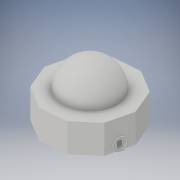
# Autodesk Inventor part: dome
Saved by Autodesk Inventor 2017 (Build 210142000, 142)
## iProperties
Created: 2018-03-05
Part Number: dome
Material: Generic
Document SubType Name: Modeling
Designer: Braxton
Density: 1 g/cm^3
Appearance: Default
Author: Braxton
Autodesk Inventor part; units mm, degrees
ref_plane "YZ Plane" through (0, 0, 0) normal (1, 0, 0) x (0, 1, 0)
sketch "Sketch1" plane through (0, 0, 0) normal (0, 1, 0) x (-1, 0, 0)
  line L0 (707.6587, -429.7359) -> (319.9155, -763.615)
  line L1 (319.9155, -763.615) -> (-190.0245, -805.8191)
  line L2 (-190.0245, -805.8191) -> (-627.3817, -540.2278)
  line L3 (-627.3817, -540.2278) -> (-825.1003, -68.2877)
  line L4 (-825.1003, -68.2877) -> (-707.6587, 429.7359)
  line L5 (-707.6587, 429.7359) -> (-319.9155, 763.615)
  line L6 (-319.9155, 763.615) -> (190.0245, 805.8191)
  line L7 (190.0245, 805.8191) -> (627.3817, 540.2278)
  line L8 (627.3817, 540.2278) -> (825.1003, 68.2877)
  line L9 (825.1003, 68.2877) -> (707.6587, -429.7359)
  point P0 (0, 0)
  point P1 (0, 0)
  dimension "d0" = 1574.8
  constraints: 20 end point, 1 coincident, 21 other
  measures "d0" distance between parallel lines of L5 L0
extrude "bace" add sketch "Sketch1" along normal blind 25.4
sketch "Sketch2" plane through (0, 25.4, 0) normal (0, 1, 0) x (1, 0, 0)
  line L0 (-319.9155, 763.615) -> (-707.6587, 429.7359) projected
  line L1 (-707.6587, 429.7359) -> (-319.9155, 763.615)
  line L2 (-319.9155, 763.615) -> (190.0245, 805.8191)
  line L3 (190.0245, 805.8191) -> (627.3817, 540.2278)
  line L4 (627.3817, 540.2278) -> (825.1003, 68.2877)
  line L5 (825.1003, 68.2877) -> (707.6587, -429.7359)
  line L6 (707.6587, -429.7359) -> (319.9155, -763.615)
  line L7 (319.9155, -763.615) -> (-190.0245, -805.8191)
  line L8 (-190.0245, -805.8191) -> (-627.3817, -540.2278)
  line L9 (-627.3817, -540.2278) -> (-825.1003, -68.2877)
  line L10 (-825.1003, -68.2877) -> (-707.6587, 429.7359)
  line L11 (-684.831, 415.8734) -> (-309.5957, 738.9822)
  line L12 (-309.5957, 738.9822) -> (183.8947, 779.825)
  line L13 (183.8947, 779.825) -> (607.1435, 522.8011)
  line L14 (607.1435, 522.8011) -> (798.4842, 66.0849)
  line L15 (798.4842, 66.0849) -> (684.831, -415.8734)
  line L16 (684.831, -415.8734) -> (309.5957, -738.9822)
  line L17 (309.5957, -738.9822) -> (-183.8947, -779.825)
  line L18 (-183.8947, -779.825) -> (-607.1435, -522.8011)
  line L19 (-607.1435, -522.8011) -> (-798.4842, -66.0849)
  line L20 (-798.4842, -66.0849) -> (-684.831, 415.8734)
  line L21 (-707.6587, 429.7359) -> (-825.1003, -68.2877) projected
  point P0 (0, 0)
  point P1 (0, 0)
  point P2 (0, 0)
  dimension "d4" = 25.4
  constraints: 40 end point, 2 coincident, 1 parallel, 42 other
  measures "d4" distance between parallel lines of L21 L20
extrude "bace wall" add sketch "Sketch2" along normal blind 508
sketch "Sketch3" plane through (0, 533.4, 0) normal (0, 1, 0) x (1, 0, 0)
  line L0 (-627.3817, -540.2278) -> (-825.1003, -68.2877) projected
  line L1 (-825.1003, -68.2877) -> (-707.6587, 429.7359)
  line L2 (-707.6587, 429.7359) -> (-319.9155, 763.615)
  line L3 (-319.9155, 763.615) -> (190.0245, 805.8191)
  line L4 (190.0245, 805.8191) -> (627.3817, 540.2278)
  line L5 (627.3817, 540.2278) -> (825.1003, 68.2877)
  line L6 (825.1003, 68.2877) -> (707.6587, -429.7359)
  line L7 (707.6587, -429.7359) -> (319.9155, -763.615)
  line L8 (319.9155, -763.615) -> (-190.0245, -805.8191)
  line L9 (-190.0245, -805.8191) -> (-627.3817, -540.2278)
  line L10 (-627.3817, -540.2278) -> (-825.1003, -68.2877)
  circle A0 centre (0, 0) radius 508
  point P0 (-798.4842, -66.0849)
  dimension "d28" = 1016
  constraints: 20 end point, 1 centre point
  measures "d28" diameter of A0
extrude "bace cieiling" add sketch "Sketch3" along normal blind 25.4
ref_plane "dome work plane" through (56.8266, 25.4, -240.9792) normal (0.9733039, 0, 0.22952) x (0.22952, 0, -0.9733039)
sketch "Sketch10" plane through (56.8266, 25.4, -240.9792) normal (0.9733039, 0, 0.22952) x (0.22952, 0, -0.9733039)
  line L0 (285.8112, 533.4) -> (260.4112, 533.4)
  line L1 (-755.5888, 533.4) -> (260.4112, 533.4) projected
  arc A0 (260.4112, 533.4) -> (-247.5888, 1041.4) centre (-247.5888, 533.4) ccw
  arc A1 (285.8112, 533.4) -> (-247.5888, 1066.8) centre (-247.5888, 533.4) ccw
  line L2 (-247.5888, 1066.8) -> (-247.5888, 1041.4)
  line L3 (-247.5888, 1041.4) -> (-247.5888, 533.4) construction
  point P0 (-247.5888, -25.4)
  dimension "d32" = 508
  dimension "d33" = 533.4
  constraints: 6 end point, 4 point on circle, 2 centre point, 2 coincident, 2 vertical, 1 midpoint
  measures "d32" radius of A0
  measures "d33" radius of A1
revolve "dome" add sketch "Sketch10" angle 360 about axis through (0, 1066.8, 0) along (0, -1, 0)
sketch "Sketch8" plane through (825.1003, 0, -68.2877) normal (0.9733039, 0, 0.22952) x (0.22952, 0, -0.9733039)
  line L0 (-255.8418, 25.4) -> (-205.0418, 25.4)
  line L1 (-205.0418, 25.4) -> (-205.0418, 194.7333)
  line L2 (-205.0418, 194.7333) -> (-255.8418, 194.7333)
  line L3 (-255.8418, 194.7333) -> (-255.8418, 25.4)
  line L4 (-255.8418, 25.4) -> (-306.6418, 25.4)
  line L5 (-306.6418, 25.4) -> (-306.6418, 194.7333)
  line L6 (-306.6418, 194.7333) -> (-255.8418, 194.7333)
  line L7 (-503.4306, 25.4) -> (-8.253, 25.4) projected
  point P0 (-255.8418, 0)
  point P1 (-255.8418, 25.4)
  dimension "d16" = 50.8
  dimension "d17" = 169.3333
  constraints: 14 end point, 2 symmetric about line, 1 horizontal, 1 midpoint, 1 perpendicular
  measures "d16" distance of L0.start L0.end
  measures "d17" distance of L0.end L1.end
extrude "door frame" cut sketch "Sketch8" against normal blind 25.4
sketch "Sketch7" plane through (825.1003, 0, -68.2877) normal (0.9733039, 0, 0.22952) x (0.22952, 0, -0.9733039)
  line L0 (-306.6418, 194.7333) -> (-205.0418, 194.7333)
  line L1 (-306.6418, 25.4) -> (-205.0418, 25.4)
  arc A0 (-198.4359, 0) -> (-313.6926, 0.2332) centre (-255.8418, 110.0667) ccw
  arc A1 (-306.6418, 194.7333) -> (-306.6418, 25.4) centre (-255.8418, 110.0667) ccw
  arc A2 (-205.0418, 25.4) -> (-205.0418, 194.7333) centre (-255.8418, 110.0667) ccw
  line L2 (-306.6418, 194.7333) -> (-205.0418, 194.7333)
  line L3 (-306.6418, 194.7333) -> (-306.6418, 25.4)
  line L4 (-313.6926, 0.2332) -> (-198.4359, 0)
  point P0 (-255.8418, 0)
  point P1 (-255.8418, 194.7333)
  point P2 (-306.6418, 110.0667)
  point P3 (-255.8418, 110.0667)
  point P4 (-256.0642, 0.1166)
  dimension "d14" = 169.3333
  dimension "d15" = 101.6
  constraints: 10 end point, 6 point on circle, 3 centre point, 3 midpoint, 2 coincident, 1 horizontal, 1 parallel
  measures "d14" distance between parallel lines of L1 L0
  measures "d15" distance of L0.start L0.end
extrude "corridor connection" add sketch "Sketch7" along normal blind 25.4
sketch "Sketch9" plane through (729.998, 25.4, 224.3381) normal (0.22952, 0, -0.9733039) x (-0.9733039, 0, -0.22952)
  line L0 (-12.7, 169.3333) -> (-6.35, 169.3333)
  line L1 (-6.35, 169.3333) -> (-6.35, 0)
  line L2 (-6.35, 0) -> (-19.05, 0)
  line L3 (-19.05, 0) -> (-19.05, 169.3333)
  line L4 (-12.7, 169.3333) -> (-19.05, 169.3333)
  line L5 (-25.4, -25.4) -> (-25.4, 208.8041) projected
  point P0 (762, -25.4)
  point P1 (-25.4, -25.4)
  point P2 (-25.4, 169.3333)
  point P3 (0, 169.3333)
  point P4 (-25.4, 0)
  point P5 (0, 0)
  point P6 (-25.4, 169.3333)
  point P7 (-25.4, -25.1668)
  dimension "d22" = 6.35
  dimension "d23" = 12.7
  dimension "d24" = 169.3333
  constraints: 10 end point, 1 point on line
  measures "d22" distance of L0.start L0.end
  measures "d23" distance of L1.end L2.end
  measures "d24" distance between parallel lines of L2 L0
extrude "left door slot" cut sketch "Sketch9" against normal blind 50.8
ref_plane "door slot mirror" through (766.3795, 25.4, 180.7241) normal (0.22952, 0, -0.9733039) x (-0.9733039, 0, -0.22952)
mirror "Mirror1" about plane through (766.3795, 25.4, 180.7241) normal (0.22952, 0, -0.9733039) of "left door slot"
body "Solid1"
